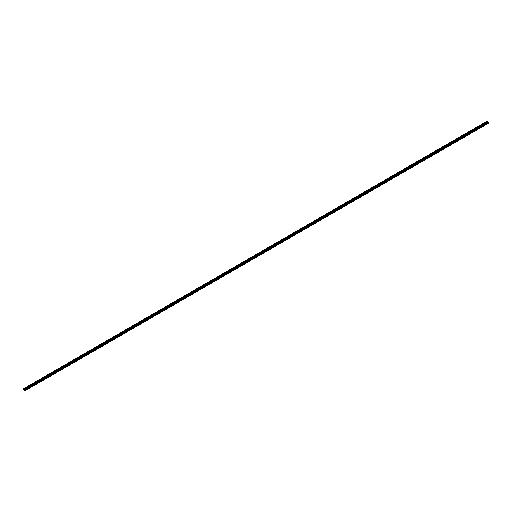
# Autodesk Inventor part: TL20240701-10100CV-DY1055
Saved by Autodesk Inventor 2022.5 (Build 265521000, 521)
## iProperties
Category: PROFILE ASSY
Manager: 호상태
Created: 2023-01-19
Part Number: TL20240701-10100CV-DY1055
User Status: 2
Material: AL6061
Description: 3
Document SubType Name: Modeling
Designer: 박성규
Density: 2.7 g/cm^3
Appearance: 알루미늄 - 평지(1)
DETAIL: Coveryor Assembly
M/C TITLE: CJ 제일제당 협동로봇 포장시스탬 PILOT 장비
PARTS NAME: Bracket
SPECIFICATION: TA20221101-CV200000-015
DocNumber: 221118_Standard_v1
Folder: .\
VDS_Category: 엔지니어링
Detail Description: Purchased products
Title: DY1055-8540L
Author: 박성규
Revision Number: A
Autodesk Inventor part; units mm, degrees
ref_plane "YZ Plane" through (0, 0, 0) normal (1, 0, 0) x (0, 1, 0)
ref_plane "XZ Plane" through (0, 0, 0) normal (0, 1, 0) x (-1, 0, 0)
ref_plane "XY Plane" through (0, 0, 0) normal (0, 0, 1) x (1, 0, 0)
sketch "스케치9" plane through (0, 0, 0) normal (0, 0, 1) x (1, 0, 0)
  line L0 (-10.2, -9) -> (-10.2, -8)
  line L1 (-10.2, -8) -> (-1.8, -8)
  line L2 (-1.8, -8) -> (-1.8, -9)
  line L3 (-1.8, -9) -> (0, -9)
  line L4 (0, -9) -> (0, 0)
  line L5 (0, 0) -> (-5.5, 0)
  line L6 (-5.5, 0) -> (-6, -1)
  line L7 (-6, -1) -> (-6.5, 0)
  line L8 (-6.5, 0) -> (-30.5, 0)
  line L9 (-30.5, 0) -> (-30.5, -2)
  line L10 (-30.5, -2) -> (-17, -2)
  line L11 (-17, -2) -> (-12, -5.0043)
  line L12 (-12, -5.0043) -> (-12, -9)
  line L13 (-12, -9) -> (-10.2, -9)
  point P0 (0, 0)
  dimension "d42" = 9
  dimension "d45" = 30.5
  constraints: 28 end point
  measures "d42" distance of L3.end L4.end
  measures "d45" distance between parallel lines of L4 L9
extrude "돌출4" add sketch "스케치9" along normal mid plane 7680
equation "\"d46\" = L1 + L2"
equation "\"L1\" = 6000"
equation "\"L2\" = 1680"
